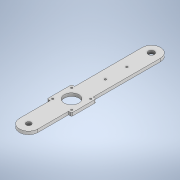
# Autodesk Inventor part: Tess
Saved by Autodesk Inventor 2022 (Build 260153000, 153)
## iProperties
Created: 2022-12-30
Part Number: Tess
Material: Generic
Document SubType Name: Modeling
Designer: nguye
Density: 1 g/cm^3
Appearance: Default
Author: nguye
Autodesk Inventor part; units mm, degrees
ref_plane "YZ Plane" through (0, 0, 0) normal (1, 0, 0) x (0, 1, 0)
ref_plane "XZ Plane" through (0, 0, 0) normal (0, 1, 0) x (-1, 0, 0)
ref_plane "XY Plane" through (0, 0, 0) normal (0, 0, 1) x (1, 0, 0)
sketch "Sketch1" plane through (0, 0, 0) normal (0, 1, 0) x (-1, 0, 0)
  circle A0 centre (0, 0) radius 15
  circle A1 centre (0, -200) radius 15
  line L0 (-15, -200) -> (-15, 0)
  line L1 (15, -200) -> (15, 0)
  line L2 (-18, -50) -> (18, -50)
  line L3 (20, -52) -> (20, -90)
  line L4 (20, -90) -> (-20, -90)
  line L5 (-20, -90) -> (-20, -52)
  line L6 (-20, -50) -> (20, -90) construction
  line L7 (20, -50) -> (-20, -90) construction
  circle A2 centre (-15.5, -85.5) radius 1.525
  circle A3 centre (-15.5, -54.5) radius 1.525
  circle A4 centre (15.5, -85.5) radius 1.525
  circle A5 centre (15.5, -54.5) radius 1.525
  circle A6 centre (0, -200) radius 5
  circle A7 centre (0, 0) radius 4
  circle A8 centre (0, -125) radius 1.5
  circle A9 centre (0, -160) radius 1.5
  arc A10 (-18, -50) -> (-20, -52) centre (-18, -52) ccw
  arc A11 (20, -52) -> (18, -50) centre (18, -52) ccw
  circle A12 centre (-18, -88) radius 2
  circle A13 centre (18, -88) radius 2
  circle A14 centre (0, -70) radius 12
  point P0 (0, -90)
  point P1 (-15, -50)
  point P2 (-20, -88)
  point P3 (-18, -90)
  point P4 (-15, -90)
  point P5 (15, -90)
  point P6 (18, -90)
  point P7 (20, -88)
  point P8 (15, -50)
  dimension "d0" = 30
  dimension "d1" = 30
  dimension "d2" = 200
  dimension "d3" = 40
  dimension "d4" = 40
  dimension "d5" = 50
  dimension "d6" = 3.05
  dimension "d7" = 3.05
  dimension "d8" = 3.05
  dimension "d9" = 3.05
  dimension "d10" = 31
  dimension "d11" = 4.5
  dimension "d12" = 4.5
  dimension "d14" = 31
  dimension "d15" = 10
  dimension "d16" = 8
  dimension "d17" = 3
  dimension "d18" = 3
  dimension "d19" = 35
  dimension "d20" = 35
  dimension "d21" = 2
  dimension "d22" = 2
  dimension "d23" = 4
  dimension "d24" = 4
  dimension "d25" = 24
  constraints: 16 end point, 15 centre point, 11 tangent, 8 point on circle, 7 vertical alignment, 4 coincident, 4 point on line, 3 midpoint, 2 horizontal alignment, 2 parallel, 1 horizontal, 1 perpendicular, 1 vertical
  measures "d0" diameter of A0
  measures "d1" diameter of A1
  measures "d2" distance of point (0, 0) A1.centre
  measures "d3" distance of L3.end L4.end
  measures "d4" distance of L7.start L3.end
  measures "d5" distance from line of point (0, 0) L2
  measures "d6" diameter of A2
  measures "d7" diameter of A3
  measures "d8" diameter of A4
  measures "d9" diameter of A5
  measures "d10" distance of A4.centre A2.centre
  measures "d11" distance from line of L5 A2.centre
  measures "d12" distance from line of L4 A2.centre
  measures "d14" distance of A5.centre A4.centre
  measures "d15" diameter of A6
  measures "d16" diameter of A7
  measures "d17" diameter of A8
  measures "d18" diameter of A9
  measures "d19" distance from line of L4 A8.centre
  measures "d20" distance of A8.centre A9.centre
  measures "d21" radius of A10
  measures "d22" radius of A11
  measures "d23" diameter of A12
  measures "d24" diameter of A13
  measures "d25" diameter of A14
extrude "Extrusion1" add sketch "Sketch1" along normal blind 5 contours A0 | L1 L2 L0 A0 | L2 A11 L3 A13 L4 L1 A4 A5 | L1 A5 A4 L4 L0 A2 A3 L2 | L0 A3 A2 L4 A12 L5 A10 L2 | A13 | A12 | L1 A1 L0 L4 | A1
body "Solid1"
